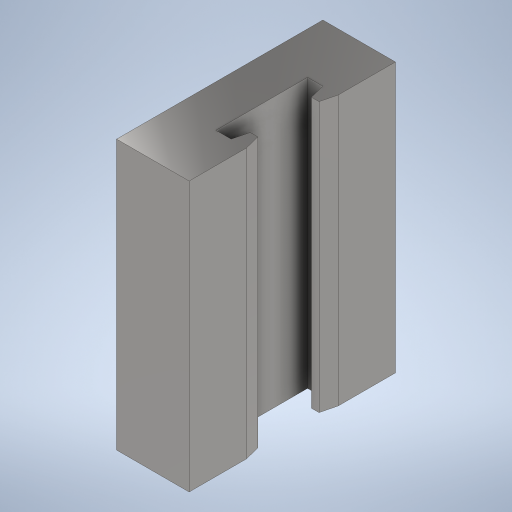
# Autodesk Inventor part: Guia trilho
Saved by Autodesk Inventor 2023 (Build 270158000, 158)
## iProperties
Created: 2023-03-23
Part Number: Guia trilho
Material: Steel, Alloy
Document SubType Name: Sheet Metal
Designer: 062190003
Density: 7.73 g/cm^3
Sheet Metal Rule: Default_mm
Appearance: Semi-Polished
Author: 062190003
Autodesk Inventor part; units mm, degrees
ref_plane "YZ Plane" through (0, 0, 0) normal (1, 0, 0) x (0, 1, 0)
ref_plane "XZ Plane" through (0, 0, 0) normal (0, 1, 0) x (-1, 0, 0)
ref_plane "XY Plane" through (0, 0, 0) normal (0, 0, 1) x (1, 0, 0)
sketch "Sketch1" plane through (0, 0, 0) normal (0, 1, 0) x (-1, 0, 0)
  line L0 (3.9616, -0.4601) -> (4.9616, -0.4601)
  line L1 (5.4616, 1.5399) -> (7.4616, 1.5399)
  line L2 (7.4616, 1.5399) -> (7.4616, -10.4601)
  line L3 (7.4616, -10.4601) -> (5.4616, -10.4601)
  line L4 (4.9616, -8.4601) -> (3.9616, -8.4601)
  line L5 (5.4616, 1.5399) -> (4.9616, -0.4601)
  line L6 (3.4616, 1.5399) -> (3.9616, -0.4601)
  line L7 (4.9616, -8.4601) -> (5.4616, -10.4601)
  line L8 (3.4616, -10.4601) -> (3.9616, -8.4601)
  line L9 (3.4616, -10.4601) -> (3.4616, -17.9601)
  line L10 (3.4616, -17.9601) -> (12.9616, -17.9601)
  line L11 (12.9616, -17.9601) -> (12.9616, 9.0399)
  line L12 (12.9616, 9.0399) -> (3.4616, 9.0399)
  line L13 (3.4616, 9.0399) -> (3.4616, 1.5399)
  point P0 (0, 0)
  point P1 (12.9616, -4.4601)
  point P2 (7.4616, -4.4601)
  point P3 (6.4616, -10.4601)
  dimension "d2" = 8
  dimension "d3" = 1
  dimension "d5" = 0.5
  dimension "d6" = 4
  dimension "d8" = 9.5
  dimension "d9" = 27
  dimension "d12" = 0
  dimension "d13" = 12
  dimension "d14" = 2
  dimension "d15" = 2
  constraints: 28 end point, 6 perpendicular, 4 equal length, 3 horizontal, 3 midpoint, 2 point on line, 1 parallel, 1 vertical
  measures "d2" distance of L0.end L4.start
  measures "d3" distance of L0.start L0.end
  measures "d5" horizontal distance of L1.start L0.end
  measures "d6" distance of L1.end L6.start
  measures "d8" distance of L9.end L10.end
  measures "d9" distance of L10.end L11.end
  measures "d12" vertical distance of point (12.962, -4.46) point (7.462, -4.46)
  measures "d13" distance of L1.end L2.end
  measures "d14" vertical distance of L6.start L0.start
  measures "d15" vertical distance of L8.start L4.end
extrude "Extrusion1" add sketch "Sketch1" along normal blind 35.25
sketch "Sketch2" plane through (-12.9616, 0, -17.9601) normal (-1, 0, 0) x (0, 0, 1)
  line L0 (0, 35.25) -> (27, 35.25) projected
  line L1 (0, 0) -> (0, 35.25) projected
  point P0 (17.9601, 0)
  point P1 (6, 27.625)
  point P2 (21, 27.625)
  point P3 (21, 7.625)
  point P4 (6, 7.625)
  dimension "d16" = 15
  dimension "d17" = 15
  dimension "d18" = 20
  dimension "d19" = 20
  dimension "d20" = 0
  dimension "d21" = 0
  dimension "d22" = 35.25
  dimension "d23" = 27
  dimension "d24" = 7.625
  dimension "d25" = 6
  measures "d16" distance of point (21, 27.625) point (6, 27.625)
  measures "d17" distance of point (21, 7.625) point (6, 7.625)
  measures "d18" distance of point (6, 7.625) point (6, 27.625)
  measures "d19" distance of point (21, 7.625) point (21, 27.625)
  measures "d20" horizontal distance of point (21, 7.625) point (21, 27.625)
  measures "d21" vertical distance of point (21, 27.625) point (6, 27.625)
  measures "d22" distance of L1.start L0.start
  measures "d23" distance of L0.start L0.end
  measures "d24" distance from line of L0 point (6, 27.625)
  measures "d25" distance from line of L1 point (6, 27.625)
hole "Hole1" at (-12.9616, 27.625, -11.9601) at (-12.9616, 27.625, 3.0399) at (-12.9616, 7.625, 3.0399) at (-12.9616, 7.625, -11.9601) direction (1, 0, 0) diameter 2.459 depth 5 tip angle 118 thread size "M3x0.5" class "6H" standard "ISO Metric profile"
equation "\"d24\" = -0.5 * d18 + 0.5 * d22"
equation "\"d25\" = -0.5 * d16 + 0.5 * d23"
equation "\"BendRadius\" = Thickness"
equation "\"BendReliefWidth\" = Thickness"
equation "\"BendReliefDepth\" = 0.5 * Thickness"
equation "\"CornerReliefSize\" = 4 * Thickness"
equation "\"MinimumRemnant\" = 2 * Thickness"
equation "\"TransitionRadius\" = BendRadius"
equation "\"JacobiRadiusSize\" = BendRadius"
equation "\"GapSize\" = Thickness"
equation "\"Thickness\" = 0.5"
body "Solid1"
